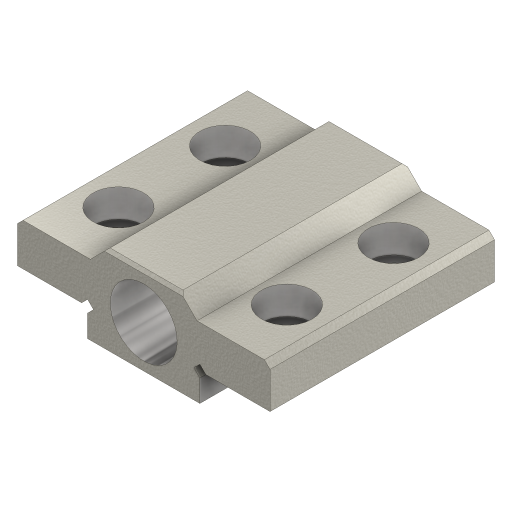
# Autodesk Inventor part: Part040. Tool Holder
Saved by Autodesk Inventor 2023.2 (Build 272271030, 271C)
## iProperties
Created: 2023-11-30
Part Number: Part040. Tool Holder
Material: Steel, Alloy
Document SubType Name: Modeling
Designer: User
Mass: 863.735 g
Surface Area: 301.113 cm^2
Volume: 111.738 cm^3
Density: 7.73 g/cm^3
Appearance: Steel - Cast
Author: User
Autodesk Inventor part; units mm, degrees
ref_plane "YZ Plane" through (0, 0, 0) normal (1, 0, 0) x (0, 1, 0)
ref_plane "XZ Plane" through (0, 0, 0) normal (0, 1, 0) x (-1, 0, 0)
ref_plane "XY Plane" through (0, 0, 0) normal (0, 0, 1) x (1, 0, 0)
sketch "Sketch1" plane through (0, 0, 0) normal (0, 0, 1) x (1, 0, 0)
  line L0 (0, 0) -> (0, 31)
  line L1 (0, 0) -> (-20, 0)
  line L2 (-20, 0) -> (-20, 7.8787)
  line L3 (-22.1213, 10) -> (-45, 10)
  line L4 (-45, 10) -> (-45, 25)
  line L5 (-45, 25) -> (-19, 25)
  line L6 (-19, 25) -> (-13, 31)
  line L7 (-13, 31) -> (0, 31)
  line L8 (-22.1213, 10) -> (-20, 12.1213)
  line L9 (-20, 12.1213) -> (-17.8787, 10)
  line L10 (-17.8787, 10) -> (-20, 7.8787)
  line L11 (0, 0) -> (20, 0)
  line L12 (20, 0) -> (20, 7.8787)
  line L13 (22.1213, 10) -> (45, 10)
  line L14 (45, 10) -> (45, 25)
  line L15 (45, 25) -> (19, 25)
  line L16 (19, 25) -> (13, 31)
  line L17 (13, 31) -> (0, 31)
  line L18 (22.1213, 10) -> (20, 12.1213)
  line L19 (20, 12.1213) -> (17.8787, 10)
  line L20 (17.8787, 10) -> (20, 7.8787)
  dimension "d0" = 31
  dimension "d1" = 10
  dimension "d2" = 15
  dimension "d3" = 45
  dimension "d4" = 3
  dimension "d5" = 38
  dimension "d6" = 90
  dimension "d7" = 40
  constraints: 42 end point, 9 symmetric about line, 7 perpendicular, 4 point on line, 2 equal length, 1 horizontal, 1 vertical
  measures "d0" distance of L0.start L0.end
  measures "d1" distance between parallel lines of L1 L3
  measures "d2" distance between parallel lines of L3 L5
  measures "d3" angle of L5 L6
  measures "d4" distance of L8.end L9.end
  measures "d5" distance of L15.end L5.end
  measures "d6" distance between parallel lines of L14 L4
  measures "d7" distance between parallel lines of L12 L2
extrude "Extrusion1" add sketch "Sketch1" along normal mid plane 80
sketch "Sketch2" plane through (0, 0, 0) normal (1, 0, 0) x (0, 1, 0)
  line L0 (15, 40) -> (15, -40)
  line L1 (15, -40) -> (25.0727, -40)
  line L2 (25.0727, -40) -> (25.0727, -34)
  line L3 (25.0727, -34) -> (26.93, 40)
  line L4 (26.93, 40) -> (15, 40)
  line L5 (0, -40) -> (0, 40) projected
  point P0 (0, 0)
  point P1 (31, 40)
  point P2 (31, -40)
  dimension "d10" = 74
  dimension "d11" = 23.86
  dimension "d12" = 1.438
  dimension "d13" = 15
  constraints: 10 end point, 2 perpendicular, 2 point on line, 1 parallel, 1 vertical
  measures "d10" vertical distance of L2.end L3.end
  measures "d11" diameter of L3.end L0
  measures "d12" angle of L0 L3
  measures "d13" distance between parallel lines of L5 L0
revolve "Revolution1" cut sketch "Sketch2" angle 360 about axis through (0, 15, 40) along (0, 0, -1)
sketch "Sketch3" plane through (19, 25, 40) normal (0, 1, 0) x (1, 0, 0)
  point P0 (-19, 40)
  point P1 (-49, 21)
  dimension "d15" = 19
  dimension "d16" = 30
  measures "d15" vertical distance of point (-49, 21) point (-19, 40)
  measures "d16" horizontal distance of point (-49, 21) point (-19, 40)
hole "Hole1" at (-30, 25, 19) direction (0, -1, 0) diameter 11 end through all counterbore diameter 18 counterbore depth 10
pattern_linear "Rectangular Pattern1" count 2 spacing 60 along (1, 0, 0) count 2 spacing 38 along (0, 0, -1) of "Hole1"
chamfer "Chamfer1" distance 2 angle 45 2 edges at (-45, 25, 0) (45, 25, 0)
chamfer "Chamfer2" distance 1 angle 45 2 edges at (0, 31, 40) (0, 31, -40)
body "Solid1"
